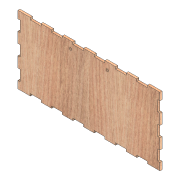
# Autodesk Inventor part: elektronica behuizing
Saved by Autodesk Inventor 2020.3 (Build 243373000, 373)
## iProperties
Created: 2020-10-19
Part Number: elektronica behuizing
Material: Wood (Birch)
Document SubType Name: Sheet Metal
Designer: Svend
Density: 0.55 g/cm^3
Sheet Metal Rule: Default_mm
Appearance: Birch - Natural Polished
Author: Svend
Autodesk Inventor part; units mm, degrees
ref_plane "YZ Plane" through (0, 0, 0) normal (1, 0, 0) x (0, 1, 0)
ref_plane "XZ Plane" through (0, 0, 0) normal (0, 1, 0) x (-1, 0, 0)
ref_plane "Work Plane1" through (0, 0, 0) normal (0, 0, 1) x (1, 0, 0)
sketch "Sketch1" plane through (0, 0, 0) normal (0, 0, 1) x (1, 0, 0)
  line L0 (0, -5) -> (43, -5) projected
  line L1 (0, -25) -> (0, -5) projected
  line L2 (0, -25) -> (3, -25) projected
  line L3 (3, -25) -> (43, -25) projected
  line L4 (43, -5) -> (43, -25) projected
  line L5 (127, -5) -> (170, -5) projected
  line L6 (127, -5) -> (127, -25) projected
  line L7 (167, -25) -> (127, -25) projected
  line L8 (170, -25) -> (167, -25) projected
  line L9 (170, -25) -> (170, -5) projected
  ellipse E0 centre (272.0385, -161.4535) end of major axis (262.0385, -161.4535) minor radius 9.7437 projected
  line L10 (264.0385, -174.9547) -> (285, -186.7467) projected
  line L11 (285, -186.7467) -> (285, -136.1602) projected
  line L12 (285, -136.1602) -> (264.0385, -147.9522) projected
  ellipse E1 centre (272.0385, -161.4535) end of major axis (256.0385, -161.4535) minor radius 15.5899 (264.0385, -147.9522) -> (264.0385, -174.9547) ccw projected
  ellipse E2 centre (-102.0385, -161.4535) end of major axis (-92.0385, -161.4535) minor radius 9.7437 projected
  line L13 (-94.0385, -174.9547) -> (-115, -186.7467) projected
  ellipse E3 centre (-102.0385, -161.4535) end of major axis (-86.0385, -161.4535) minor radius 15.5899 (-94.0385, -174.9547) -> (-94.0385, -147.9522) ccw projected
  line L14 (-115, -136.1602) -> (-94.0385, -147.9522) projected
  line L15 (-115, -186.7467) -> (-115, -136.1602) projected
  line L16 (-115, -136.1602) -> (-115, -5) construction
  line L17 (-115, -5) -> (285, -5) construction
  line L18 (285, -5) -> (285, -186.7467) construction
  line L19 (285, -186.7467) -> (-115, -186.7467) construction
  line L20 (-115, -186.7467) -> (-115, -136.1602) construction
  line L21 (285, -5) -> (-115, -5)
  line L22 (-115, -5) -> (-115, -186.7467)
  line L23 (-115, -186.7467) -> (285, -186.7467)
  line L24 (285, -186.7467) -> (285, -5)
  circle A0 centre (147, -15) radius 3.25
  circle A1 centre (23, -15) radius 3.25
  circle A2 centre (23, -15) radius 2.4585 projected
  circle A3 centre (147, -15) radius 2.4585 projected
  line L25 (-115, -5) -> (285, -5)
  line L26 (285, -5) -> (285, 5)
  line L27 (285, 5) -> (-115, 5)
  line L28 (-115, 5) -> (-115, -5)
  point P0 (0, 0)
  point P1 (170, -15)
  point P2 (147, -25)
  point P3 (23, -25)
  point P4 (43, -15)
  dimension "d0" = 6.5
  dimension "d2" = 10
  constraints: 26 end point, 5 equal length, 5 perpendicular, 4 midpoint, 2 centre point, 2 collinear, 2 horizontal, 2 horizontal alignment, 2 vertical alignment, 1 equal radius, 1 point on line, 1 vertical, 3 other
  measures "d0" diameter of A1
  measures "d2" distance between parallel lines of L21 L27
extrude "Plate1" add sketch "Sketch1" along normal blind 6 contours L21 L28 L27 L26 L5 L0 | L0 L4 L3 L2 L1 | L1 L2 L3 L4 L21 L6 L7 L8 L9 L24 L12 E1 L10 L23 L13 E3 L14 L22 | L5 L9 L8 L7 L6 | L14 E3 L13 L15 | L10 E1 L12 L11 | E0 | E2 | A0 | A1 | A2 | A3
sketch "Sketch2" plane through (0, 0, 6) normal (0, 0, 1) x (1, 0, 0)
  line L0 (-115, -186.7467) -> (-115, 5) projected
  line L1 (285, -186.7467) -> (-115, -186.7467) projected
  line L2 (285, 5) -> (285, -186.7467) projected
  line L3 (-115, 5) -> (285, 5) projected
  line L4 (285, -186.7467) -> (285, 5) projected
  line L5 (285, -75.8734) -> (279, -75.8734)
  line L6 (279, -75.8734) -> (279, -105.8734)
  line L7 (279, -105.8734) -> (285, -105.8734)
  line L8 (285, -105.8734) -> (285, -75.8734)
  line L9 (285, -45.8734) -> (279, -45.8734)
  line L10 (279, -45.8734) -> (279, -15.8734)
  line L11 (279, -15.8734) -> (285, -15.8734)
  line L12 (285, -15.8734) -> (285, -45.8734)
  line L13 (285, -135.8734) -> (279, -135.8734)
  line L14 (279, -135.8734) -> (279, -165.8734)
  line L15 (279, -165.8734) -> (285, -165.8734)
  line L16 (285, -165.8734) -> (285, -135.8734)
  line L17 (285, 5) -> (-115, 5) construction
  line L18 (85, 5) -> (85, -186.7467) construction
  line L19 (-115, -75.8734) -> (-109, -75.8734)
  line L20 (-109, -75.8734) -> (-109, -105.8734)
  line L21 (-109, -105.8734) -> (-115, -105.8734)
  line L22 (-115, -105.8734) -> (-115, -75.8734)
  line L23 (-115, -45.8734) -> (-109, -45.8734)
  line L24 (-109, -45.8734) -> (-109, -15.8734)
  line L25 (-109, -15.8734) -> (-115, -15.8734)
  line L26 (-115, -15.8734) -> (-115, -45.8734)
  line L27 (-115, -135.8734) -> (-109, -135.8734)
  line L28 (-109, -135.8734) -> (-109, -165.8734)
  line L29 (-109, -165.8734) -> (-115, -165.8734)
  line L30 (-115, -165.8734) -> (-115, -135.8734)
  line L31 (-115, -186.7467) -> (285, -186.7467) projected
  line L32 (250, -186.7467) -> (220, -186.7467)
  line L33 (220, -186.7467) -> (220, -180.7467)
  line L34 (220, -180.7467) -> (250, -180.7467)
  line L35 (250, -180.7467) -> (250, -186.7467)
  line L36 (190, -186.7467) -> (160, -186.7467)
  line L37 (160, -186.7467) -> (160, -180.7467)
  line L38 (160, -180.7467) -> (190, -180.7467)
  line L39 (190, -180.7467) -> (190, -186.7467)
  line L40 (130, -186.7467) -> (100, -186.7467)
  line L41 (100, -186.7467) -> (100, -180.7467)
  line L42 (100, -180.7467) -> (130, -180.7467)
  line L43 (130, -180.7467) -> (130, -186.7467)
  line L44 (285, -90.8734) -> (-115, -90.8734) construction
  line L45 (250, 5) -> (220, 5)
  line L46 (220, 5) -> (220, -1)
  line L47 (220, -1) -> (250, -1)
  line L48 (250, -1) -> (250, 5)
  line L49 (190, 5) -> (160, 5)
  line L50 (160, 5) -> (160, -1)
  line L51 (160, -1) -> (190, -1)
  line L52 (190, -1) -> (190, 5)
  line L53 (130, 5) -> (100, 5)
  line L54 (100, 5) -> (100, -1)
  line L55 (100, -1) -> (130, -1)
  line L56 (130, -1) -> (130, 5)
  circle A0 centre (23, -15) radius 3.25
  line L57 (-80, -186.7467) -> (-50, -186.7467)
  line L58 (-50, -186.7467) -> (-50, -180.7467)
  line L59 (-50, -180.7467) -> (-80, -180.7467)
  line L60 (-80, -180.7467) -> (-80, -186.7467)
  line L61 (-20, -186.7467) -> (10, -186.7467)
  line L62 (10, -186.7467) -> (10, -180.7467)
  line L63 (10, -180.7467) -> (-20, -180.7467)
  line L64 (-20, -180.7467) -> (-20, -186.7467)
  line L65 (40, -186.7467) -> (70, -186.7467)
  line L66 (70, -186.7467) -> (70, -180.7467)
  line L67 (70, -180.7467) -> (40, -180.7467)
  line L68 (40, -180.7467) -> (40, -186.7467)
  line L69 (70, 5) -> (70, -1)
  line L70 (40, 5) -> (70, 5)
  line L71 (40, -1) -> (40, 5)
  line L72 (10, 5) -> (10, -1)
  line L73 (-20, 5) -> (10, 5)
  line L74 (10, -1) -> (-20, -1)
  line L75 (-20, -1) -> (-20, 5)
  line L76 (70, -1) -> (40, -1)
  line L77 (-50, 5) -> (-50, -1)
  line L78 (-80, 5) -> (-50, 5)
  line L79 (-80, -1) -> (-80, 5)
  line L80 (-50, -1) -> (-80, -1)
  point P0 (0, 0)
  point P1 (115, -180.7467)
  point P2 (115, -1)
  point P3 (55, -180.7467)
  point P4 (55, -1)
  dimension "d3" = 6
  dimension "d4" = 30
  dimension "d5" = 30
  dimension "d6" = 30
  dimension "d7" = 30
  dimension "d8" = 30
  dimension "d10" = 15
  constraints: 148 end point, 53 symmetric about line, 16 point on line, 12 parallel, 7 equal length, 7 horizontal, 6 midpoint, 6 perpendicular, 1 centre point, 1 coincident
  measures "d3" distance of L7.end L6.end
  measures "d4" distance of L6.end L5.end
  measures "d5" distance between parallel lines of L5 L9
  measures "d6" distance between parallel lines of L7 L13
  measures "d7" distance between parallel lines of L43 L37
  measures "d8" distance from line of L36.start L33
  measures "d10" distance between parallel lines of L18 L41
extrude "Cut1" cut sketch "Sketch2" against normal blind 6 contours L0 L27 L28 L29 | L60 L59 L58 L1 | L0 L19 L20 L21 | L64 L63 L62 L1 | L0 L25 L24 L23 | L68 L67 L66 L1 | L41 L42 L43 L1 | L3 L77 L80 L79 | L37 L38 L39 L1 | L3 L72 L74 L75 | L33 L34 L35 L1 | L3 L69 L76 L71 | L3 L56 L55 L54 | L15 L14 L13 L2 | L3 L52 L51 L50 | L7 L6 L5 L2 | L3 L48 L47 L46 | L9 L10 L11 L2
sketch "Sketch3" plane through (0, 0, 0) normal (0, 0, -1) x (-1, 0, 0)
  circle A0 centre (-147, -15) radius 3.25 projected
  circle A1 centre (-23, -15) radius 3.25 projected
  circle A2 centre (-136.75, -15) radius 3.25
  circle A3 centre (-33.25, -15) radius 3.25
  line L0 (115, -5) -> (-285, -5) construction
  line L1 (-136.75, -15) -> (-33.25, -15) construction
  point P0 (0, 0)
  point P1 (-23, -15)
  point P2 (-85, -15)
  point P3 (-85, -5)
  dimension "d13" = 103.5
  constraints: 2 centre point, 2 end point, 2 equal radius, 2 horizontal alignment, 2 midpoint, 1 horizontal, 1 vertical alignment
  measures "d13" distance of L1.start L1.end
extrude "Cut2" cut sketch "Sketch3" against normal blind 6 contours A2 | A3
equation "\"d5\" = d4"
equation "\"d6\" = d5"
equation "\"d7\" = d4"
equation "\"d8\" = d7"
equation "\"d11\" = Thickness"
equation "\"d14\" = Thickness"
equation "\"d1\" = Thickness"
equation "\"BendRadius\" = Thickness"
equation "\"BendReliefWidth\" = Thickness"
equation "\"BendReliefDepth\" = 0.5 * Thickness"
equation "\"CornerReliefSize\" = 4 * Thickness"
equation "\"MinimumRemnant\" = 2 * Thickness"
equation "\"TransitionRadius\" = BendRadius"
equation "\"JacobiRadiusSize\" = BendRadius"
equation "\"GapSize\" = Thickness"
equation "\"Thickness\" = 6"
body "Solid1"
